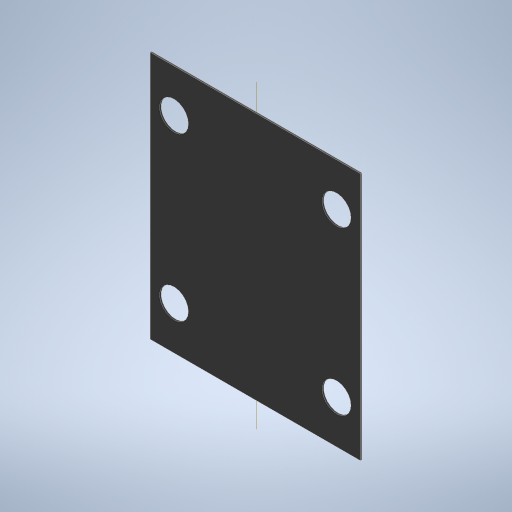
# Autodesk Inventor part: board_setter_safety
Saved by Autodesk Inventor 2024.1 (Build 281209000, 209)
## iProperties
Created: 2024-10-09
Part Number: board_setter_safety
Material: 一般
Document SubType Name: モデリング
Designer: hibik
Density: 1 g/cm^3
Appearance: 既定
Author: hibik
Autodesk Inventor part; units mm, degrees
ref_plane "YZ Plane" through (0, 0, 0) normal (1, 0, 0) x (0, 1, 0)
ref_plane "XZ Plane" through (0, 0, 0) normal (0, 1, 0) x (-1, 0, 0)
ref_plane "XY Plane" through (0, 0, 0) normal (0, 0, 1) x (1, 0, 0)
sketch "スケッチ1" plane through (0, 0, 0) normal (0, 0, 1) x (1, 0, 0)
  line L0 (-22, -24) -> (22, -24)
  line L1 (22, -24) -> (22, 24)
  line L2 (22, 24) -> (-22, 24)
  line L3 (-22, 24) -> (-22, -24)
  line L4 (-22, -24) -> (22, 24) construction
  line L5 (22, -24) -> (-22, 24) construction
  line L6 (-17, 15) -> (17, 15)
  line L7 (17, 15) -> (17, -19)
  line L8 (17, -19) -> (-17, -19)
  line L9 (-17, -19) -> (-17, 15)
  circle A0 centre (-17, 15) radius 3
  circle A1 centre (17, 15) radius 3
  circle A2 centre (17, -19) radius 3
  circle A3 centre (-17, -19) radius 3
  circle A4 centre (-17, 15) radius 8
  circle A5 centre (17, 15) radius 8
  circle A6 centre (17, -19) radius 8
  circle A7 centre (-17, -19) radius 8
  line L10 (-22, -24) -> (22, -24)
  line L11 (22, -24) -> (22, -28)
  line L12 (22, -28) -> (-22, -28)
  line L13 (-22, -28) -> (-22, -24)
  line L14 (-2.5, 15) -> (2.5, 15)
  line L15 (2.5, 15) -> (2.5, -19)
  line L16 (2.5, -19) -> (-2.5, -19)
  line L17 (-2.5, -19) -> (-2.5, 15)
  line L18 (10.5, 15) -> (10.5, -19)
  line L19 (5.5, -19) -> (5.5, 15)
  line L20 (18.5, 15) -> (18.5, -19)
  line L21 (13.5, -19) -> (13.5, 15)
  line L22 (-5.5, 15) -> (-5.5, -19)
  line L23 (-10.5, -19) -> (-10.5, 15)
  line L24 (2.5, 15) -> (2.5, -19)
  line L25 (-2.5, -19) -> (-2.5, 15)
  line L26 (10.5, 15) -> (10.5, -19)
  line L27 (5.5, -19) -> (5.5, 15)
  line L28 (-13.5, 15) -> (-13.5, -19)
  line L29 (-18.5, -19) -> (-18.5, 15)
  line L30 (-5.5, 15) -> (-5.5, -19)
  line L31 (-10.5, -19) -> (-10.5, 15)
  line L32 (2.5, 15) -> (2.5, -19)
  line L33 (-2.5, -19) -> (-2.5, 15)
  point P0 (0, 0)
  point P1 (-9, 15)
  point P2 (9, 15)
  point P3 (17, 7)
  point P4 (17, -11)
  point P5 (9, -19)
  point P6 (-9, -19)
  point P7 (-17, -11)
  point P8 (-17, 7)
  point P9 (22, -24)
  point P10 (0, 15)
  point P11 (-18.5, 7.1419)
  point P12 (-18.5, -11.1419)
  point P13 (-13.5, -11.8063)
  point P14 (-13.5, 7.8063)
  point P15 (-10.5, 15)
  point P16 (-10.5, -19)
  point P17 (-5.5, -19)
  point P18 (-5.5, 15)
  point P19 (13.5, 7.8063)
  point P20 (13.5, -11.8063)
  point P21 (18.5, -11.1419)
  point P22 (18.5, 7.1419)
  point P23 (5.5, 15)
  point P24 (5.5, -19)
  point P25 (10.5, -19)
  point P26 (10.5, 15)
  point P27 (-2.5, -19)
  point P28 (2.5, 15)
  point P29 (-10.5, -14.3363)
  point P30 (-10.5, 10.3363)
  point P31 (10.5, 10.3363)
  point P32 (10.5, -14.3363)
  dimension "d0" = 48
  dimension "d1" = 44
  dimension "d2" = 34
  dimension "d3" = 5
  dimension "d4" = 5
  dimension "d5" = 6
  dimension "d6" = 16
  dimension "d11" = 4
  dimension "d12" = 5
  dimension "d15" = 8
  dimension "d18" = 8
  measures "d0" distance of L2.end L0.start
  measures "d1" distance of L1.end L2.end
  measures "d2" distance of L7.end L8.end
  measures "d3" distance between parallel lines of L3 L9
  measures "d4" distance between parallel lines of L0 L8
  measures "d5" diameter of A0
  measures "d6" diameter of A4
  measures "d11" distance of L10.end L11.end
  measures "d12" distance between parallel lines of L15 L17
  measures "d15" distance of L14.end L18.start
  measures "d18" distance of L14.end L22.start
extrude "プレート1" add sketch "スケッチ1" along normal blind 1.5 contours L3 A7 L29 A3 L8 L0 | L0 A7 L13 | A7 L8 A6 L0 | L0 A6 L11 L12 L13 A7 | L3 A4 L29 A7 | A6 L8 A2 L20 L1 L0 | L0 L11 A6 | L8 L23 A7 | L3 A4 L6 A0 L29 | A7 L9 A3 L29 | A6 L18 L8 | L22 L6 L17 L8 | L8 L28 A7 L23 | A7 L28 A4 L23 | L3 L2 L1 A5 L6 A4 | L29 A0 L9 A4 | A7 L28 L8 A3 L9 | A6 L20 A5 L1 | L18 A6 L21 L8 | L8 L15 L6 L19 | L18 A5 L21 A6 | L23 L6 A4 | A4 L28 L6 L23 | L9 A0 L6 L28 A4 | A5 L20 A1 L6 L1 | L20 A2 L7 A6 | L21 A6 L7 A2 L8 | L18 L6 L21 A5 | A5 L6 L18 | A5 L7 A1 L20 | L21 L6 A1 L7 A5
sketch "スケッチ2" plane through (0, 0, 1.5) normal (0, 0, 1) x (1, 0, 0)
  line L0 (11.5, -21.5) -> (11.5, -14.8) projected
  line L1 (11.5, -21.5) -> (12, -21.5) projected
  line L2 (12, -21.5) -> (12, -24) projected
  line L3 (18, -24) -> (14, -24) projected
  line L4 (18, -14) -> (18, -24) construction
  line L5 (12.3, -14) -> (18, -14) projected
  circle A0 centre (12.3, -14.8) radius 0.8
  circle A1 centre (14, -23.2) radius 0.8
  line L6 (0, 0) -> (0, -10)
  circle A2 centre (-12.3, -14.8) radius 0.8
  circle A3 centre (-14, -23.2) radius 0.8
  arc A4 (11.5, -14.8) -> (12.3, -14) centre (12.3, -14.8) ccw projected
  line L7 (14, -24) -> (12, -24) projected
  circle A5 centre (14, -23.2) radius 0.8 projected
  dimension "d21" = 1.6
  dimension "d22" = 1.6
  dimension "d25" = 2
  constraints: 4 centre point, 3 tangent, 2 end point, 2 symmetric about line, 1 vertical, 1 vertical alignment, 2 other
  measures "d21" diameter of A0
  measures "d22" diameter of A1
  measures "d25" distance from line of L2 A1.centre
extrude "切り取り1" cut sketch "スケッチ2" against normal blind 1.5
sketch "スケッチ3" plane through (0, 0, 1.5) normal (0, 0, 1) x (1, 0, 0)
  circle A0 centre (0, 19) radius 0.8
  circle A1 centre (-10, 19) radius 0.8
  circle A2 centre (10, 19) radius 0.8
  line L0 (-22, 24) -> (22, 24) projected
  point P0 (0, 0)
  point P1 (0, 24)
  dimension "d26" = 1.6
  dimension "d27" = 1.6
  dimension "d28" = 1.6
  dimension "d29" = 5
  dimension "d30" = 10
  dimension "d31" = 10
  constraints: 3 centre point, 2 horizontal alignment, 1 midpoint, 1 vertical alignment
  measures "d26" diameter of A0
  measures "d27" diameter of A1
  measures "d28" diameter of A2
  measures "d29" distance from line of L0 A0.centre
  measures "d30" distance of A1.centre A0.centre
  measures "d31" distance of A2.centre A0.centre
extrude "切り取り2" cut sketch "スケッチ3" against normal blind 1.5
sketch "スケッチ5" plane through (0, 0, 1.5) normal (0, 0, 1) x (1, 0, 0)
  line L0 (-32.0708, 30) -> (50, 30)
  line L1 (50, 30) -> (50, -40)
  line L2 (50, -40) -> (-32.0708, -40)
  line L3 (-32.0708, -40) -> (-32.0708, 30)
  point P0 (0, 0)
  constraints: 8 end point, 2 parallel, 1 horizontal, 1 perpendicular
extrude "押し出し2" cut sketch "スケッチ5" against normal blind 1.2
sketch "スケッチ6" plane through (0, 0, 0.3) normal (0, 0, 1) x (1, 0, 0)
  circle A0 centre (-10, 19) radius 0.8 projected
  circle A1 centre (0, 19) radius 0.8 projected
  circle A2 centre (10, 19) radius 0.8 projected
  circle A3 centre (-12.3, -14.8) radius 0.8 projected
  circle A4 centre (12.3, -14.8) radius 0.8 projected
  circle A5 centre (14, -23.2) radius 0.8 projected
  circle A6 centre (-14, -23.2) radius 0.8 projected
  line L0 (13.5, 7.8063) -> (13.5, -11.8063) projected
  arc A7 (13.5, 7.8063) -> (18.5, 7.1419) centre (17, 15) ccw projected
  line L1 (18.5, -11.1419) -> (18.5, 7.1419) projected
  arc A8 (18.5, -11.1419) -> (13.5, -11.8063) centre (17, -19) ccw projected
  arc A9 (-13.5, -11.8063) -> (-18.5, -11.1419) centre (-17, -19) ccw projected
  line L2 (-18.5, 7.1419) -> (-18.5, -11.1419) projected
  arc A10 (-18.5, 7.1419) -> (-13.5, 7.8063) centre (-17, 15) ccw projected
  line L3 (-13.5, -11.8063) -> (-13.5, 7.8063) projected
  arc A11 (10.5, -14.3363) -> (9, -19) centre (17, -19) ccw projected
  line L4 (5.5, -19) -> (9, -19) projected
  line L5 (5.5, 15) -> (5.5, -19) projected
  line L6 (9, 15) -> (5.5, 15) projected
  arc A12 (9, 15) -> (10.5, 10.3363) centre (17, 15) ccw projected
  line L7 (10.5, -14.3363) -> (10.5, 10.3363) projected
  circle A13 centre (-17, 15) radius 3 projected
  circle A14 centre (-17, -19) radius 3 projected
  line L8 (-2.5, -19) -> (2.5, -19) projected
  line L9 (-2.5, 15) -> (-2.5, -19) projected
  line L10 (2.5, 15) -> (-2.5, 15) projected
  line L11 (2.5, -19) -> (2.5, 15) projected
  circle A15 centre (17, -19) radius 3 projected
  circle A16 centre (17, 15) radius 3 projected
  line L12 (-9, -19) -> (-5.5, -19) projected
  arc A17 (-9, -19) -> (-10.5, -14.3363) centre (-17, -19) ccw projected
  line L13 (-10.5, 10.3363) -> (-10.5, -14.3363) projected
  arc A18 (-10.5, 10.3363) -> (-9, 15) centre (-17, 15) ccw projected
  line L14 (-5.5, 15) -> (-9, 15) projected
  line L15 (-5.5, -19) -> (-5.5, 15) projected
  line L16 (-22, 24) -> (22, 24) projected
  line L17 (-22, -28) -> (-22, 24) projected
  line L18 (22, -28) -> (-22, -28) projected
  line L19 (22, 24) -> (22, -28) projected
  point P0 (0, 0)
extrude "押し出し3" add sketch "スケッチ6" against normal up to surface (0.3 mm away) contours A0 | A1 | A2 | A3 | A4 | A5 | A6 | A7 L1 A8 L0 | A9 L2 A10 L3 | A11 L4 L5 L6 A12 L7 | L9 L10 L11 L8 | A17 L13 A18 L14 L15 L12
equation "\"d4\" = d3"
equation "\"d23\" = Thickness"
equation "\"d32\" = Thickness"
equation "\"d10\" = Thickness"
equation "\"BendRadius\" = Thickness"
equation "\"BendReliefWidth\" = Thickness"
equation "\"BendReliefDepth\" = 0.5 * Thickness"
equation "\"CornerReliefSize\" = 4 * Thickness"
equation "\"MinimumRemnant\" = 2 * Thickness"
equation "\"TransitionRadius\" = BendRadius"
equation "\"JacobiRadiusSize\" = BendRadius"
equation "\"GapSize\" = Thickness"
equation "\"Thickness\" = 1.5"
